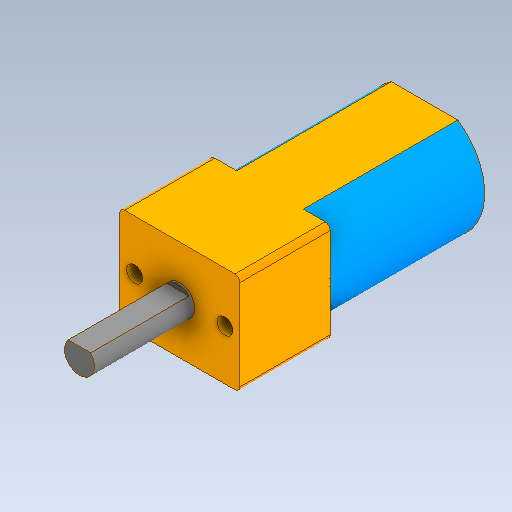
# Autodesk Inventor part: n20
Saved by Autodesk Inventor 2020 (Build 240168000, 168)
## iProperties
Created: 2020-09-25
Part Number: n20
Material: Generic
Document SubType Name: Modeling
Designer: alnwlsn
Density: 1 g/cm^3
Appearance: Default
Author: alnwlsn
Autodesk Inventor part; units mm, degrees
ref_plane "YZ Plane" through (0, 0, 0) normal (1, 0, 0) x (0, 1, 0)
ref_plane "XZ Plane" through (0, 0, 0) normal (0, 1, 0) x (-1, 0, 0)
ref_plane "XY Plane" through (0, 0, 0) normal (0, 0, 1) x (1, 0, 0)
sketch "Sketch1" plane through (0, 0, 0) normal (0, 0, 1) x (1, 0, 0)
  line L0 (0, 0) -> (12, 0)
  line L1 (12, 0) -> (12, 10)
  line L2 (12, 10) -> (0, 10)
  line L3 (0, 10) -> (0, 0)
  line L4 (6, 10) -> (6, 0) construction
  line L5 (1.5, 5) -> (10.5, 5) construction
  circle A0 centre (1.5, 5) radius 0.8
  circle A1 centre (10.5, 5) radius 0.8
  circle A2 centre (6, 5) radius 1.5
  dimension "d0" = 10
  dimension "d1" = 12
  dimension "d2" = 9
  dimension "d3" = 1.6
  dimension "d4" = 3
  constraints: 12 end point, 4 midpoint, 3 centre point, 3 coincident, 2 parallel, 2 perpendicular, 1 equal radius, 1 horizontal
  measures "d0" distance of L2.end L0.start
  measures "d1" distance of L1.end L2.end
  measures "d2" distance of L5.start L5.end
  measures "d3" diameter of A1
  measures "d4" diameter of A2
extrude "Extrusion1" add sketch "Sketch1" against normal blind 9 contours L3 L2 L1 L0 | A0 | A1 | A2
extrude "Extrusion2" cut sketch "Sketch1" against normal through all contours A0 | A1
extrude "Extrusion3" add sketch "Sketch1" along normal blind 10 contours A2
sketch "Sketch2" plane through (6, 5, 10) normal (0, 0, 1) x (1, 0, 0)
  circle A0 centre (0, 0) radius 1.5 projected
  circle A1 centre (0, 0) radius 1.5 projected
  line L0 (-1.118, 1) -> (1.118, 1)
  point P0 (-6, -5)
  point P1 (-1.118, 1)
  point P2 (1.118, 1)
  dimension "d11" = 1
  constraints: 2 end point, 2 point on circle, 1 horizontal
  measures "d11" distance from line of A0.centre L0
extrude "Extrusion4" cut sketch "Sketch2" against normal blind 9.8 contours L0 A0 picked at (-0.0599, 1.1631)
sketch "Sketch3" plane through (0, 0, -9) normal (0, 0, -1) x (-1, 0, 0)
  circle A0 centre (-6, 5) radius 1.5 projected
  circle A1 centre (-6, 5) radius 6
  circle A2 centre (-10.5, 5) radius 0.8 projected
  circle A3 centre (-1.5, 5) radius 0.8 projected
  line L0 (-12, 0) -> (0, 0) projected
  line L1 (0, 0) -> (0, 10) projected
  line L2 (0, 10) -> (-12, 10) projected
  line L3 (-12, 10) -> (-12, 0) projected
  point P0 (-2.6834, 10)
  point P1 (-9.3166, 10)
  point P2 (-9.3166, 0)
  point P3 (-2.6834, 0)
  constraints: 1 centre point, 1 coincident, 1 tangent
extrude "Extrusion5" add sketch "Sketch3" along normal blind 15.4 contours A0 | A1 L0 L2 | A2 | A3
sketch "Sketch4" plane through (0, 0, -24.4) normal (0, 0, -1) x (-1, 0, 0)
  arc A0 (-2.6834, 0) -> (-2.6834, 10) centre (-6, 5) ccw projected
  circle A1 centre (-6, 5) radius 2.5
  point P0 (0, 0)
  dimension "d16" = 5
  constraints: 1 centre point, 1 coincident
  measures "d16" diameter of A1
extrude "Extrusion6" add sketch "Sketch4" along normal blind 0.8
fillet "Fillet1" radius 0.5 4 edges at (12, 10, -4.5) (0, 10, -4.5) (12, 0, -4.5) (0, 0, -4.5)
body "Solid1"
